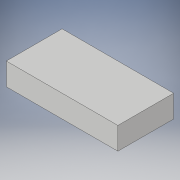
# Autodesk Inventor part: EpoxyFiberMountBase
Saved by Autodesk Inventor 2019 (Build 230136000, 136)
## iProperties
Created: 2019-05-24
Part Number: EpoxyFiberMountBase
Material: Generic
Document SubType Name: Modeling
Designer: aorfi
Density: 1 g/cm^3
Appearance: Default
Author: aorfi
Autodesk Inventor part; units mm, degrees
ref_plane "YZ Plane" through (0, 0, 0) normal (1, 0, 0) x (0, 1, 0)
ref_plane "XZ Plane" through (0, 0, 0) normal (0, 1, 0) x (-1, 0, 0)
ref_plane "XY Plane" through (0, 0, 0) normal (0, 0, 1) x (1, 0, 0)
sketch "Sketch1" plane through (0, 0, 0) normal (0, 1, 0) x (-1, 0, 0)
  line L0 (-5, 2.5) -> (5, 2.5)
  line L1 (5, 2.5) -> (5, -2.5)
  line L2 (5, -2.5) -> (-5, -2.5)
  line L3 (-5, -2.5) -> (-5, 2.5)
  line L4 (-5, 2.5) -> (5, -2.5) construction
  line L5 (5, 2.5) -> (-5, -2.5) construction
  point P0 (0, 0)
  dimension "d0" = 5
  dimension "d1" = 10
  constraints: 12 end point, 2 midpoint, 2 parallel, 1 horizontal, 1 perpendicular
  measures "d0" distance of L0.end L1.end
  measures "d1" distance of L0.start L0.end
extrude "Extrusion1" add sketch "Sketch1" along normal mid plane 2
body "Solid1"
